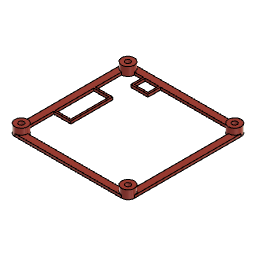
UnoHolder (Autodesk Fusion 360 design; units mm, degrees)
Autodesk Fusion 360 part; units mm, degrees
note: some values were not read from the file. Set by a fixed rule: which sketch regions a step uses.
sketch "Sketch1" plane through (0, 0, 0) normal (0, 0, 1) x (1, 0, 0)
  line L0 (7.5, 0) -> (132.5, 0)
  line L1 (140, 7.5) -> (140, 132.5)
  line L2 (132.5, 140) -> (7.5, 140)
  line L3 (0, 132.5) -> (0, 7.5)
  circle A0 centre (7.5, 132.5) radius 7.5
  circle A1 centre (7.5, 132.5) radius 3
  line L4 (0, 70) -> (140, 70) construction
  line L5 (70, 140) -> (70, 0) construction
  circle A2 centre (7.5, 7.5) radius 3
  circle A3 centre (7.5, 7.5) radius 7.5
  circle A4 centre (132.5, 132.5) radius 7.5
  circle A5 centre (132.5, 132.5) radius 3
  circle A6 centre (132.5, 7.5) radius 3
  circle A7 centre (132.5, 7.5) radius 7.5
  line L6 (7.5, 7.5) -> (132.5, 7.5)
  line L7 (132.5, 7.5) -> (132.5, 132.5)
  line L8 (132.5, 132.5) -> (7.5, 132.5)
  line L9 (7.5, 132.5) -> (7.5, 7.5)
  line L10 (7.5, 92.5) -> (25.5, 92.5)
  line L11 (25.5, 92.5) -> (25.5, 47.5)
  line L12 (25.5, 47.5) -> (7.5, 47.5)
  line L13 (7.5, 47.5) -> (7.5, 92.5)
  line L14 (7.5, 70) -> (25.5, 70) construction
  line L15 (7.5, 94.5) -> (27.5, 94.5)
  line L16 (27.5, 94.5) -> (27.5, 45.5)
  line L17 (27.5, 45.5) -> (7.5, 45.5)
  line L18 (7.5, 45.5) -> (7.5, 94.5)
  line L19 (7.5, 70) -> (27.5, 70) construction
  line L20 (27.5, 132.5) -> (43.5, 132.5)
  line L21 (43.5, 132.5) -> (43.5, 119.9)
  line L22 (43.5, 119.9) -> (27.5, 119.9)
  line L23 (27.5, 119.9) -> (27.5, 132.5)
  line L24 (25.5, 132.5) -> (45.5, 132.5)
  line L25 (45.5, 132.5) -> (45.5, 117.9)
  line L26 (45.5, 117.9) -> (25.5, 117.9)
  line L27 (25.5, 117.9) -> (25.5, 132.5)
  line L28 (35.5, 119.9) -> (35.5, 122) construction
  line L29 (35.5, 117.9) -> (35.5, 122) construction
  dimension "d3" = 15
  dimension "d4" = 6
  dimension "d6" = 140
  dimension "d7" = 140
  dimension "d10" = 45
  dimension "d11" = 18
  dimension "d12" = 49
  dimension "d13" = 20
  dimension "d14" = 16
  dimension "d15" = 12.6
  dimension "d16" = 20
  dimension "d17" = 20
  dimension "d18" = 14.6
  constraint horizontal L0
  constraint vertical L1
  constraint horizontal L2
  constraint vertical L3
  constraint concentric A0 A1
  constraint tangent L2 A0
  constraint tangent L3 A0
  constraint coincident A0 L2.end
  constraint coincident L2 L5.start
  constraint coincident A0 L3.start
  constraint coincident L3 L4.start
  constraint symmetric A0 L4 A3
  constraint symmetric A1 L4 A2
  constraint symmetric A0 L5 A4
  constraint symmetric A1 L5 A5
  constraint symmetric L5 A2 A6
  constraint symmetric L5 A3 A7
  constraint coincident A4 L2.start
  constraint coincident A4 L1.end
  constraint coincident L1 L4.end
  constraint coincident A7 L0.end
  constraint coincident L0 L5.end
  constraint coincident A7 L1.start
  constraint coincident A3 L3.end
  constraint coincident A3 L0.start
  constraint coincident origin L3
  constraint coincident origin L0
  constraint horizontal L6
  constraint vertical L7
  constraint horizontal L8
  constraint vertical L9
  constraint coincident A4.centre A5.centre
  constraint coincident A2.centre A3.centre
  constraint horizontal L10
  constraint vertical L11
  constraint horizontal L12
  constraint vertical L13
  constraint midpoint L13 L14.start
  constraint midpoint L11 L14.end
  constraint coincident A2.centre L13
  constraint coincident L4.start L14
  constraint horizontal L15
  constraint vertical L16
  constraint horizontal L17
  constraint vertical L18
  constraint midpoint L18 L14.start
  constraint midpoint L16 L19.end
  constraint coincident A2.centre L18
  constraint coincident L4.start L19
  constraint horizontal L20
  constraint vertical L21
  constraint horizontal L22
  constraint vertical L23
  constraint coincident A0.centre L20
  constraint horizontal L24
  constraint vertical L25
  constraint horizontal L26
  constraint vertical L27
  constraint coincident A0.centre L24
  constraint midpoint L22 L28.start
  constraint perpendicular L22 L28
  constraint midpoint L26 L29.start
  constraint perpendicular L26 L29
  constraint coincident L28.end L29.end
  measures "d3" diameter of A0
  measures "d4" diameter of A1
  measures "d6" distance of L1 L3
  measures "d7" distance of L0 L2
  measures "d10" distance of L10.end L11.end
  measures "d11" distance of L10.start L10.end
  measures "d12" distance of L15.end L16.end
  measures "d13" distance of L15.start L15.end
  measures "d14" distance of L21.end L22.end
  measures "d15" distance of L20.end L21.end
  measures "d16" distance of L9 L23
  measures "d17" distance of L25.end L26.end
  measures "d18" distance of L24.end L25.end
extrude "Extrude1" add sketch "Sketch1" along normal blind 10 contours A2 A3 L6 L9 | A6 A7 L6 L7 | A2 A3 L6 L9 | A6 A7 L6 L7 | A0 A1 L8 L9 | A4 A5 L7 L8 | A0 A1 L8 L9 | A4 A5 L7 L8 makes body 1 at (14.9627, 6.7532, 3.3333) makes body 2 at (139.9627, 8.2468, 6.6667) makes body 3 at (14.8513, 133.9861, 3.3333) makes body 4 at (139.4111, 135.4133, 6.6667)
extrude "Extrude1'" add sketch "Sketch1" along normal blind 3 separate body contours L0 A3 A7 L6 | A2 A3 L6 L9 | A6 A7 L6 L7 | L3 A0 A3 L9 L13 L18 | A2 A3 L6 L9 | L1 A4 A7 L7 | A6 A7 L6 L7 | A0 A1 L8 L9 | A4 A5 L7 L8 | L2 A0 A4 L8 L20 L24 | A0 A1 L8 L9 | L9 L10 L11 L12 L15 L16 L17 L18 | A4 A5 L7 L8 | L8 L21 L22 L23 L24 L25 L26 L27 makes body 5 in component "Component"
combine "Combine1" operation add target body 4 tool bodies 5
combine "Combine2" operation add target body 2 tool bodies 4
combine "Combine3" operation add target body 1 tool bodies 2
combine "Combine4" operation add target body 3 tool bodies 1
component "Component" placed x (1, 0, 0) y (0, 1, 0) z (0, 0, 1) at (0, 0, 0)
equation "d1 = 140 mm"
equation "d2 = d1"
equation "d18 = d15 + 2 mm"
